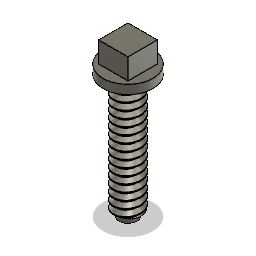
Screw (Autodesk Fusion 360 design; units mm, degrees)
Autodesk Fusion 360 part; units mm, degrees
sketch "Sketch1" plane through (0, 0, 0) normal (0, 1, 0) x (1, 0, 0)
  line L0 (0.3125, 0.3125) -> (-0.3125, 0.3125)
  line L1 (-0.3125, 0.3125) -> (-0.3125, -0.3125)
  line L2 (-0.3125, -0.3125) -> (0.3125, -0.3125)
  line L3 (0.3125, -0.3125) -> (0.3125, 0.3125)
  line L4 (0.3125, 0.3125) -> (-0.3125, -0.3125) construction
  line L5 (-0.3125, 0.3125) -> (0.3125, -0.3125) construction
  dimension "d1" = 0.625
  dimension "d2" = 0.625
extrude "Extrude1" add sketch "Sketch1" along normal blind 0.44
sketch "Sketch2" plane through (0, 0, 0) normal (0, -1, 0) x (1, 0, 0)
  line L0 (0.3125, -0.3125) -> (0.3125, 0.3125)
  line L1 (0.3125, 0.3125) -> (-0.3125, 0.3125)
  line L2 (-0.3125, 0.3125) -> (-0.3125, -0.3125)
  line L3 (-0.3125, -0.3125) -> (0.3125, -0.3125)
  circle A0 centre (0, 0) radius 0.53
  dimension "d5" = 1.06
  measures "d5" diameter of A0
extrude "Extrude2" add sketch "Sketch2" along normal blind 0.19 contours L0 L1 L2 L3 | A0
sketch "Sketch3" plane through (0, -0.19, 0) normal (0, -1, 0) x (1, 0, 0)
  circle A0 centre (0, 0) radius 0.19
  circle A1 centre (0, 0) radius 0.53
  dimension "d9" = 0.38
  measures "d9" diameter of A0
sketch "Sketch5" plane through (0, -0.19, 0) normal (0, -1, 0) x (1, 0, 0)
  circle A0 centre (0, 0) radius 0.53
  circle A1 centre (0, 0) radius 0.3
  dimension "d17" = 0.6
  measures "d17" diameter of A1
extrude "Extrude5" add sketch "Sketch5" along normal blind 2.5 contours A1
sketch "Sketch6" plane through (0, -2.69, 0) normal (0, -1, 0) x (1, 0, 0)
  circle A0 centre (0, 0) radius 0.19
  circle A1 centre (0, 0) radius 0.3
  dimension "d21" = 0.38
  measures "d21" diameter of A0
extrude "Extrude6" add sketch "Sketch6" along normal blind 0.1 contours A0
thread "Thread2" "ANSI Metric M Profile 0.6 M0.6x0.15 6g" major diameter 0.588 minor diameter 0.404 pitch 0.15 angle 60 modelled right hand crest width 0.0187 on face at (0.2996, -1.8567, -0.015) crest through (0.294, -0.1806, 0)
